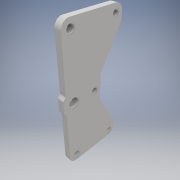
# Autodesk Inventor part: Balancim_3-Cabos_Modelo1
Saved by Autodesk Inventor 2018 (Build 220112000, 112)
## iProperties
Created: 2021-04-28
Part Number: Balancim_3-Cabos_Modelo1
Material: Generic
Document SubType Name: Modeling
Designer: l01767
Density: 1 g/cm^3
Appearance: Default
Author: l01767
Autodesk Inventor part; units mm, degrees
ref_plane "YZ Plane" through (0, 0, 0) normal (1, 0, 0) x (0, 1, 0)
ref_plane "XZ Plane" through (0, 0, 0) normal (0, 1, 0) x (-1, 0, 0)
ref_plane "XY Plane" through (0, 0, 0) normal (0, 0, 1) x (1, 0, 0)
sketch "Sketch1" plane through (0, 0, 0) normal (1, 0, 0) x (0, 1, 0)
  circle A0 centre (45, 0) radius 11
  line L0 (45, 0) -> (0, 0)
  circle A1 centre (130, 235) radius 11
  line L1 (73.2002, 0) -> (73.2002, 46.6199)
  line L2 (77.2194, 61.6199) -> (155.9808, 198.0385)
  line L3 (160, 213.0385) -> (160, 235)
  arc A2 (160, 235) -> (130, 265) centre (130, 235) ccw
  line L4 (130, 235) -> (130, 265) construction
  line L5 (130, 235) -> (160, 235) construction
  line L6 (130, 265) -> (-45, 265)
  circle A3 centre (-45, 0) radius 18
  line L7 (0, 0) -> (0, 265)
  circle A4 centre (-45, 235) radius 13
  arc A5 (-45, 265) -> (-75, 235) centre (-45, 235) ccw
  line L8 (-45, 235) -> (-75, 235) construction
  line L9 (-45, 235) -> (-45, 265) construction
  line L10 (-75, 235) -> (-75, 39.1421)
  line L11 (0, 0) -> (-45, 0)
  circle A6 centre (130, -235) radius 11
  line L12 (73.2002, 0) -> (73.2002, -46.6199)
  line L13 (77.2194, -61.6199) -> (155.9808, -198.0385)
  line L14 (160, -213.0385) -> (160, -235)
  arc A7 (130, -265) -> (160, -235) centre (130, -235) ccw
  line L15 (130, -265) -> (-45, -265)
  circle A8 centre (-45, -235) radius 13
  arc A9 (-75, -235) -> (-45, -265) centre (-45, -235) ccw
  line L16 (-45, -235) -> (-75, -235) construction
  line L17 (-75, -235) -> (-75, -39.1421)
  arc A10 (155.9808, 198.0385) -> (160, 213.0385) centre (130, 213.0385) ccw
  arc A11 (77.2194, 61.6199) -> (73.2002, 46.6199) centre (103.2002, 46.6199) ccw
  arc A12 (73.2002, -46.6199) -> (77.2194, -61.6199) centre (103.2002, -46.6199) ccw
  arc A13 (160, -213.0385) -> (155.9808, -198.0385) centre (130, -213.0385) ccw
  line L18 (-77.9289, 32.0711) -> (-82.0711, 27.9289)
  line L19 (-85, 20.8579) -> (-85, 0)
  line L20 (-77.9289, -32.0711) -> (-82.0711, -27.9289)
  line L21 (-85, -20.8579) -> (-85, 0)
  arc A14 (-77.9289, 32.0711) -> (-75, 39.1421) centre (-85, 39.1421) ccw
  arc A15 (-82.0711, 27.9289) -> (-85, 20.8579) centre (-75, 20.8579) ccw
  arc A16 (-85, -20.8579) -> (-82.0711, -27.9289) centre (-75, -20.8579) ccw
  arc A17 (-75, -39.1421) -> (-77.9289, -32.0711) centre (-85, -39.1421) ccw
  point P0 (73.2002, 54.6584)
  point P1 (160, 205)
  point P2 (-75, -35)
  point P3 (48.2002, -10.5242)
  point P4 (73.2002, -54.6584)
  point P5 (160, -205)
  point P6 (-85, 25)
  point P7 (-75, 35)
  point P8 (-85, -25)
  dimension "d0" = 22
  dimension "d1" = 22
  dimension "d2" = 470
  dimension "d3" = 90
  dimension "d4" = 36
  dimension "d7" = 30
  dimension "d8" = 26
  dimension "d9" = 90
  dimension "d11" = 25
  dimension "d12" = 85
  dimension "d13" = 90
  dimension "d14" = 30
  dimension "d15" = 30
  dimension "d16" = 30
  dimension "d19" = 45
  dimension "d20" = 40
  dimension "d21" = 50
  dimension "d22" = 10
  constraints: 44 end point, 24 point on circle, 18 tangent, 17 centre point, 17 point on line, 12 symmetric about line, 7 equal radius, 5 vertical, 4 coincident, 3 horizontal, 2 horizontal alignment, 1 collinear, 1 vertical alignment, 7 other
  measures "d1" diameter of A1
  measures "d2" diameter of A1.centre L0
  measures "d3" angle of L5 L4
  measures "d4" diameter of A3
  measures "d7" radius of A2
  measures "d8" diameter of A4
  measures "d9" angle of L9 L8
  measures "d11" distance from line of L1 point (48.2, -10.524)
  measures "d12" horizontal distance of A1.centre L0.start
  measures "d13" distance of L0.start L11.end
  measures "d14" angle of L1 L2
  measures "d15" distance of point (160, 205) L3.end
  measures "d16" radius of A10
  measures "d19" angle of L10 L18
  measures "d20" distance from line of L11.end L19
  measures "d21" diameter of point (-85, 25) L11
  measures "d22" radius of A14
extrude "Extrusion1" add sketch "Sketch1" along normal mid plane 25.4
body "Solid1"
